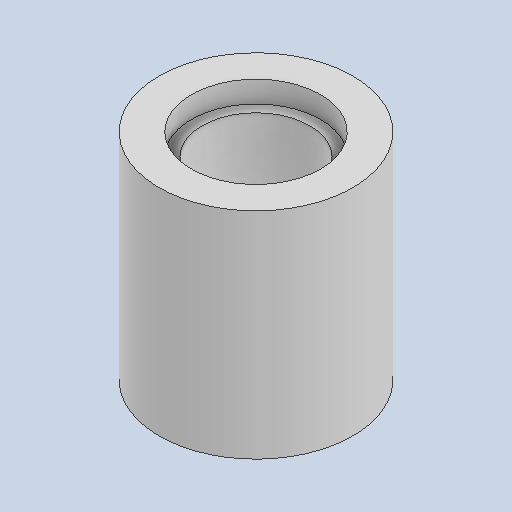
# Autodesk Inventor part: Link
Saved by Autodesk Inventor 2025.3 (Build 293356030, 356C)
## iProperties
Created: 2025-09-07
Part Number: Link
Material: 일반
Document SubType Name: Modeling
Designer: MSI
Density: 1 g/cm^3
Appearance: 기본값
Author: MSI
Autodesk Inventor part; units mm, degrees
ref_plane "YZ Plane" through (0, 0, 0) normal (1, 0, 0) x (0, 1, 0)
ref_plane "XZ Plane" through (0, 0, 0) normal (0, 1, 0) x (-1, 0, 0)
ref_plane "XY Plane" through (0, 0, 0) normal (0, 0, 1) x (1, 0, 0)
sketch "스케치1" plane through (0, 0, 0) normal (0, 1, 0) x (-1, 0, 0)
  circle A0 centre (0, 0) radius 45
  dimension "d0" = 90
  constraints: 1 centre point, 1 coincident
  measures "d0" diameter of A0
extrude "돌출1" add sketch "스케치1" along normal mid plane 100
sketch "스케치2" plane through (0, 50, 0) normal (0, 1, 0) x (1, 0, 0)
  circle A0 centre (0, 0) radius 45 projected
  constraints: 1 coincident
hole "구멍1" at (0, 50, 0) direction (0, -1, 0) diameter 50 end through all counterbore diameter 60 counterbore depth 10
